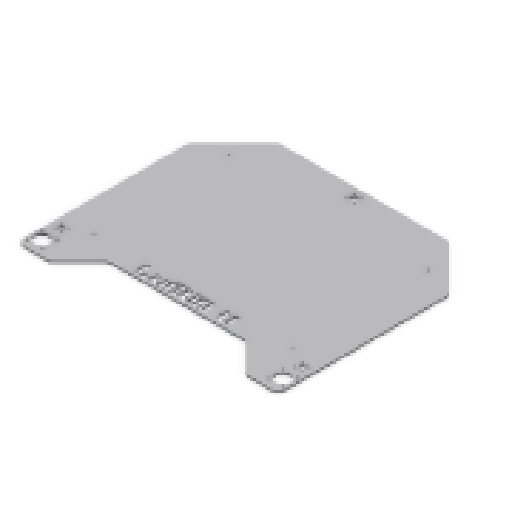
# Autodesk Inventor part: Z Axis Base
Saved by Autodesk Inventor 2023.2 (Build 272271000, 271)
## iProperties
Created: 2023-02-02
Part Number: Z Axis Base
Material: Aluminum 6061
Document SubType Name: Modeling
Designer: remop
Density: 2.7 g/cm^3
Appearance: Aluminum - Dark
Author: remop
Autodesk Inventor part; units mm, degrees
ref_plane "YZ Plane" through (0, 0, 0) normal (1, 0, 0) x (0, 1, 0)
ref_plane "XZ Plane" through (0, 0, 0) normal (0, 1, 0) x (-1, 0, 0)
ref_plane "XY Plane" through (0, 0, 0) normal (0, 0, 1) x (1, 0, 0)
sketch "Sketch1" plane through (0, 0, 0) normal (0, 1, 0) x (-1, 0, 0)
  circle A0 centre (158.2314, 130.3812) radius 11.25 projected
  circle A1 centre (158.2314, 160.3812) radius 6 projected
  circle A2 centre (-213.7686, 130.3812) radius 11.25 projected
  circle A3 centre (-213.7686, 160.3812) radius 6 projected
  circle A4 centre (-27.7686, -135.6188) radius 11 projected
  circle A5 centre (125.7314, 112.8812) radius 1.75
  circle A6 centre (125.7314, -96.1188) radius 1.75
  circle A7 centre (-181.2686, -96.1188) radius 1.75
  circle A8 centre (-181.2686, 112.8812) radius 1.75
  line L0 (222.2314, 188.3812) -> (-277.7686, 188.3812) projected
  line L1 (222.2314, -171.6188) -> (-277.7686, -171.6188) projected
  line L2 (174.2314, 183.3812) -> (124.2314, 183.3812)
  line L3 (124.2314, 183.3812) -> (78.7314, 137.8812)
  line L4 (78.7314, 137.8812) -> (-134.2686, 137.8812)
  line L5 (-134.2686, 137.8812) -> (-179.7686, 183.3812)
  line L6 (-179.7686, 183.3812) -> (-229.7686, 183.3812)
  line L7 (-229.7686, 183.3812) -> (-229.7686, -151.6188)
  line L8 (-229.7686, -151.6188) -> (174.2314, -151.6188)
  line L9 (174.2314, -151.6188) -> (174.2314, 183.3812)
  line L10 (222.2314, -171.6188) -> (222.2314, 188.3812) projected
  line L11 (-277.7686, 188.3812) -> (-277.7686, -171.6188) projected
  circle A9 centre (-213.7686, 160.3812) radius 11.5
  circle A10 centre (-225.2686, 171.8812) radius 2.1
  circle A11 centre (-202.2686, 171.8812) radius 2.1
  circle A12 centre (-202.2686, 148.8812) radius 2.1
  circle A13 centre (-225.2686, 148.8812) radius 2.1
  circle A14 centre (158.2314, 160.3812) radius 11.5
  circle A15 centre (146.7314, 171.8812) radius 2.1
  circle A16 centre (169.7314, 171.8812) radius 2.1
  circle A17 centre (169.7314, 148.8812) radius 2.1
  circle A18 centre (146.7314, 148.8812) radius 2.1
  circle A19 centre (-213.7686, 130.3812) radius 4.5
  circle A20 centre (-219.2686, 124.8812) radius 1.6
  circle A21 centre (-219.2686, 135.8812) radius 1.6
  circle A22 centre (-208.2686, 135.8812) radius 1.6
  circle A23 centre (-208.2686, 124.8812) radius 1.6
  circle A24 centre (158.2314, 130.3812) radius 4.5
  circle A25 centre (152.7314, 135.8812) radius 1.6
  circle A26 centre (163.7314, 135.8812) radius 1.6
  circle A27 centre (163.7314, 124.8812) radius 1.6
  circle A28 centre (152.7314, 124.8812) radius 1.6
  circle A29 centre (-27.7686, -135.6188) radius 4.5
  circle A30 centre (-33.2686, -130.1188) radius 1.6
  circle A31 centre (-22.2686, -130.1188) radius 1.6
  circle A32 centre (-22.2686, -141.1188) radius 1.6
  circle A33 centre (-33.2686, -141.1188) radius 1.6
  point P0 (0, 0)
  point P1 (149.2314, 183.3812)
  dimension "d0" = 307
  dimension "d1" = 209
  dimension "d2" = 3.5
  dimension "d3" = 153.5
  dimension "d4" = 360
  dimension "d5" = 75.5
  dimension "d6" = 5
  dimension "d7" = 48
  dimension "d8" = 20
  dimension "d9" = 48
  dimension "d10" = 5
  dimension "d12" = 45
  dimension "d13" = 50
  dimension "d14" = 45
  dimension "d15" = 25
  dimension "d18" = 23
  dimension "d19" = 11.5
  dimension "d20" = 11.5
  dimension "d21" = 11.5
  dimension "d22" = 11.5
  dimension "d23" = 4.2
  dimension "d24" = 11.5
  dimension "d25" = 11.5
  dimension "d26" = 11.5
  dimension "d27" = 11.5
  dimension "d28" = 9
  dimension "d29" = 5.5
  dimension "d30" = 5.5
  dimension "d31" = 5.5
  dimension "d32" = 5.5
  dimension "d33" = 3.2
  dimension "d35" = 5.5
  dimension "d36" = 5.5
  dimension "d37" = 5.5
  dimension "d39" = 5.5
  dimension "d40" = 5.5
  dimension "d41" = 5.5
  dimension "d42" = 5.5
  dimension "d43" = 5.5
  constraints: 29 centre point, 24 equal radius, 16 end point, 12 horizontal alignment, 12 vertical alignment, 5 coincident, 3 parallel, 1 collinear, 1 horizontal, 1 midpoint, 1 perpendicular
  measures "d0" distance of A8.centre A5.centre
  measures "d1" distance of A6.centre A5.centre
  measures "d2" diameter of A5
  measures "d3" horizontal distance of A6.centre A4.centre
  measures "d4" distance between parallel lines of L1 L0
  measures "d5" distance from line of L1 A7.centre
  measures "d6" distance between parallel lines of L0 L6
  measures "d7" distance between parallel lines of L11 L7
  measures "d8" distance between parallel lines of L1 L8
  measures "d9" distance between parallel lines of L10 L9
  measures "d10" distance from line of L0 point (149.231, 183.381)
  measures "d12" angle of L2 L3
  measures "d13" distance of L2.start L2.end
  measures "d14" angle of L6 L5
  measures "d15" distance from line of A5.centre L4
  measures "d18" diameter of A9
  measures "d19" horizontal distance of A3.centre A10.centre
  measures "d20" horizontal distance of A3.centre A11.centre
  measures "d21" horizontal distance of A10.centre A9.centre
  measures "d22" horizontal distance of A13.centre A3.centre
  measures "d23" diameter of A13
  measures "d24" horizontal distance of A15.centre A1.centre
  measures "d25" horizontal distance of A18.centre A1.centre
  measures "d26" horizontal distance of A1.centre A18.centre
  measures "d27" horizontal distance of A17.centre A14.centre
  measures "d28" diameter of A19
  measures "d29" horizontal distance of A21.centre A2.centre
  measures "d30" horizontal distance of A19.centre A21.centre
  measures "d31" horizontal distance of A22.centre A2.centre
  measures "d32" horizontal distance of A20.centre A2.centre
  measures "d33" diameter of A20
  measures "d35" horizontal distance of A25.centre A0.centre
  measures "d36" horizontal distance of A25.centre A0.centre
  measures "d37" horizontal distance of A0.centre A26.centre
  measures "d39" horizontal distance of A0.centre A28.centre
  measures "d40" horizontal distance of A31.centre A29.centre
  measures "d41" horizontal distance of A30.centre A4.centre
  measures "d42" horizontal distance of A31.centre A29.centre
  measures "d43" horizontal distance of A32.centre A29.centre
extrude "Extrusion1" add sketch "Sketch1" along normal blind 3 contours A0 | A2 | A4 | L9 L8 L7 L6 L5 L4 L3 L2
sketch "Sketch2" plane through (0, 3, 0) normal (0, 1, 0) x (1, 0, 0)
  line L0 (-124.2314, -183.3812) -> (-78.7314, -137.8812) projected
  line L1 (-78.7314, -137.8812) -> (134.2686, -137.8812) projected
  line L2 (134.2686, -137.8812) -> (179.7686, -183.3812) projected
  line L3 (179.7686, -183.3812) -> (229.7686, -183.3812) projected
  line L4 (229.7686, -183.3812) -> (229.7686, 151.6188) projected
  line L5 (229.7686, 151.6188) -> (-174.2314, 151.6188) projected
  line L6 (-174.2314, 151.6188) -> (-174.2314, -183.3812) projected
  line L7 (-174.2314, -183.3812) -> (-124.2314, -183.3812) projected
  circle A0 centre (-158.2314, -130.3812) radius 4.5 projected
  circle A1 centre (-152.7314, -135.8812) radius 1.6 projected
  circle A2 centre (-163.7314, -135.8812) radius 1.6 projected
  circle A3 centre (-163.7314, -124.8812) radius 1.6 projected
  circle A4 centre (-152.7314, -124.8812) radius 1.6 projected
  circle A5 centre (213.7686, -130.3812) radius 4.5 projected
  circle A6 centre (219.2686, -124.8812) radius 1.6 projected
  circle A7 centre (219.2686, -135.8812) radius 1.6 projected
  circle A8 centre (208.2686, -135.8812) radius 1.6 projected
  circle A9 centre (208.2686, -124.8812) radius 1.6 projected
  circle A10 centre (27.7686, 135.6188) radius 4.5 projected
  circle A11 centre (33.2686, 130.1188) radius 1.6 projected
  circle A12 centre (22.2686, 130.1188) radius 1.6 projected
  circle A13 centre (22.2686, 141.1188) radius 1.6 projected
  circle A14 centre (33.2686, 141.1188) radius 1.6 projected
  circle A15 centre (-125.7314, -112.8812) radius 1.75 projected
  circle A16 centre (-125.7314, 96.1188) radius 1.75 projected
  circle A17 centre (181.2686, 96.1188) radius 1.75 projected
  circle A18 centre (181.2686, -112.8812) radius 1.75 projected
  circle A19 centre (-146.7314, -148.8812) radius 2.1 projected
  circle A20 centre (-169.7314, -148.8812) radius 2.1 projected
  circle A21 centre (-169.7314, -171.8812) radius 2.1 projected
  circle A22 centre (-146.7314, -171.8812) radius 2.1 projected
  circle A23 centre (-158.2314, -160.3812) radius 11.5 projected
  circle A24 centre (225.2686, -148.8812) radius 2.1 projected
  circle A25 centre (202.2686, -148.8812) radius 2.1 projected
  circle A26 centre (202.2686, -171.8812) radius 2.1 projected
  circle A27 centre (225.2686, -171.8812) radius 2.1 projected
  circle A28 centre (213.7686, -160.3812) radius 11.5 projected
  line L8 (-71.2064, -116.1262) -> (126.7436, -116.1262) construction
  line L9 (126.7436, -116.1262) -> (126.7436, -129.6362) construction
  line L10 (126.7436, -129.6362) -> (-71.2064, -129.6362) construction
  line L11 (-71.2064, -129.6362) -> (-71.2064, -116.1262) construction
  line L12 (-41.9641, -132.872) -> (-44.5632, -130.2729)
  line L13 (-44.5632, -130.2729) -> (-44.5632, -112.872)
  line L14 (-44.5632, -112.872) -> (-37.5955, -112.872)
  line L15 (-37.5955, -112.872) -> (-37.5955, -132.872)
  line L16 (-37.5955, -132.872) -> (-41.9641, -132.872)
  line L17 (-36.7844, -132.872) -> (-36.7844, -126.9549)
  line L18 (-36.7844, -126.9549) -> (-23.66, -126.9549)
  line L19 (-23.66, -126.9549) -> (-23.66, -132.872)
  line L20 (-23.66, -132.872) -> (-36.7844, -132.872)
  line L21 (-9.3743, -132.8536) -> (-19.3282, -132.8536)
  line L22 (-19.3282, -132.8536) -> (-22.554, -129.6277)
  line L23 (-22.554, -129.6277) -> (-22.554, -118.4388)
  line L24 (-22.554, -118.4388) -> (-15.4941, -118.4388)
  line L25 (-15.4941, -118.4388) -> (-15.4941, -126.9365)
  line L26 (-15.4941, -126.9365) -> (-9.3743, -126.9365)
  line L27 (-9.3743, -126.9365) -> (-9.3743, -132.8536)
  line L28 (-1.5402, -132.8536) -> (-8.6001, -132.8536)
  line L29 (-8.6001, -132.8536) -> (-8.6001, -118.4388)
  line L30 (-8.6001, -118.4388) -> (-1.5402, -118.4388)
  line L31 (-1.5402, -118.4388) -> (-1.5402, -132.8536)
  line L32 (6.5889, -132.872) -> (2.1649, -132.872)
  line L33 (2.1649, -132.872) -> (-0.4342, -130.2729)
  line L34 (-0.4342, -130.2729) -> (-0.4342, -115.4711)
  line L35 (-0.4342, -115.4711) -> (2.1649, -112.872)
  line L36 (2.1649, -112.872) -> (6.5889, -112.872)
  line L37 (6.5889, -112.872) -> (6.5889, -132.872)
  line L38 (20.5797, -119.0471) -> (7.3999, -119.0471)
  line L39 (7.3999, -119.0471) -> (7.3999, -112.872)
  line L40 (7.3999, -112.872) -> (20.5797, -112.872)
  line L41 (20.5797, -112.872) -> (20.5797, -119.0471)
  line L42 (20.5797, -132.872) -> (7.3999, -132.872)
  line L43 (7.3999, -132.872) -> (7.3999, -126.9549)
  line L44 (7.3999, -126.9549) -> (20.5797, -126.9549)
  line L45 (20.5797, -126.9549) -> (20.5797, -132.872)
  line L46 (20.5797, -124.7061) -> (7.3999, -124.7061)
  line L47 (7.3999, -124.7061) -> (7.3999, -119.8582)
  line L48 (7.3999, -119.8582) -> (20.5797, -119.8582)
  line L49 (20.5797, -119.8582) -> (20.5797, -124.7061)
  line L50 (34.8654, -132.8904) -> (28.3216, -132.8904)
  line L51 (28.3216, -132.8904) -> (21.6856, -126.2545)
  line L52 (21.6856, -126.2545) -> (21.6856, -112.872)
  line L53 (21.6856, -112.872) -> (28.7455, -112.872)
  line L54 (28.7455, -112.872) -> (28.7455, -126.5678)
  line L55 (28.7455, -126.5678) -> (34.8654, -126.5678)
  line L56 (34.8654, -126.5678) -> (34.8654, -132.8904)
  line L57 (35.6396, -132.872) -> (35.6396, -112.872)
  line L58 (35.6396, -112.872) -> (42.5889, -112.872)
  line L59 (42.5889, -112.872) -> (42.5889, -126.2176)
  line L60 (42.5889, -126.2176) -> (35.6396, -132.872)
  line L61 (50.7548, -132.872) -> (46.2939, -132.872)
  line L62 (46.2939, -132.872) -> (43.6949, -130.2729)
  line L63 (43.6949, -130.2729) -> (43.6949, -115.4711)
  line L64 (43.6949, -115.4711) -> (46.3124, -112.872)
  line L65 (46.3124, -112.872) -> (56.8746, -112.872)
  line L66 (56.8746, -112.872) -> (56.8746, -119.0471)
  line L67 (56.8746, -119.0471) -> (50.7548, -119.0471)
  line L68 (50.7548, -119.0471) -> (50.7548, -132.872)
  line L69 (64.7087, -130.2545) -> (62.0912, -132.872)
  line L70 (62.0912, -132.872) -> (51.4921, -132.872)
  line L71 (51.4921, -132.872) -> (51.4921, -126.9549)
  line L72 (51.4921, -126.9549) -> (57.6488, -126.9549)
  line L73 (57.6488, -126.9549) -> (57.6488, -112.872)
  line L74 (57.6488, -112.872) -> (62.0912, -112.872)
  line L75 (62.0912, -112.872) -> (64.7087, -115.4895)
  line L76 (64.7087, -115.4895) -> (64.7087, -130.2545)
  line L77 (92.9299, -132.8904) -> (86.3861, -132.8904)
  line L78 (86.3861, -132.8904) -> (79.7502, -126.2545)
  line L79 (79.7502, -126.2545) -> (79.7502, -112.872)
  line L80 (79.7502, -112.872) -> (86.8101, -112.872)
  line L81 (86.8101, -112.872) -> (86.8101, -126.5678)
  line L82 (86.8101, -126.5678) -> (92.9299, -126.5678)
  line L83 (92.9299, -126.5678) -> (92.9299, -132.8904)
  line L84 (93.7041, -132.872) -> (93.7041, -112.872)
  line L85 (93.7041, -112.872) -> (100.6534, -112.872)
  line L86 (100.6534, -112.872) -> (100.6534, -126.2176)
  line L87 (100.6534, -126.2176) -> (93.7041, -132.872)
  point P0 (0, 0)
  point P1 (27.7686, -116.1262)
  point P2 (-71.2064, -122.8812)
  dimension "d44" = 15
  constraints: 2 midpoint, 1 vertical alignment, 2 other
  measures "d44" distance from line of L1 point (-71.206, -122.881)
extrude "Extrusion2" cut sketch "Sketch2" against normal through all contours L12 L13 L14 L15 L16 | L17 L18 L19 L20 | L21 L22 L23 L24 L25 L26 L27 | L28 L29 L30 L31 | L32 L33 L34 L35 L36 L37 | L38 L39 L40 L41 | L42 L43 L44 L45 | L46 L47 L48 L49 | L50 L51 L52 L53 L54 L55 L56 | L57 L58 L59 L60 | L61 L62 L63 L64 L65 L66 L67 L68 | L69 L70 L71 L72 L73 L74 L75 L76 | L77 L78 L79 L80 L81 L82 L83 | L84 L85 L86 L87
sketch "Sketch3" plane through (0, 3, 0) normal (0, 1, 0) x (1, 0, 0)
  line L0 (134.2686, -137.8812) -> (179.7686, -183.3812) projected
  line L1 (229.7686, -183.3812) -> (229.7686, 151.6188) projected
  line L2 (229.7686, 151.6188) -> (-174.2314, 151.6188) projected
  line L3 (-174.2314, 151.6188) -> (-174.2314, -183.3812) projected
  line L4 (-124.2314, -183.3812) -> (-78.7314, -137.8812) projected
  line L5 (-103.5207, 151.6188) -> (-174.2314, 80.9081)
  line L6 (-174.2314, 151.6188) -> (-174.2314, -183.3812) projected
  line L7 (229.7686, 80.9081) -> (159.0579, 151.6188)
  point P0 (0, 0)
  point P1 (-174.2314, 80.9081)
  dimension "d47" = 100
  constraints: 4 end point, 4 point on line, 2 parallel, 1 perpendicular
  measures "d47" distance of L7.start L7.end
extrude "Extrusion3" cut sketch "Sketch3" against normal through all
fillet "Fillet1" radius 10 10 edges at (-174.2314, 1.5, 183.3812) (-124.2314, 1.5, 183.3812) (229.7686, 1.5, 183.3812) (179.7686, 1.5, 183.3812) (134.2686, 1.5, 137.8812) (229.7686, 1.5, -80.9081) (159.0579, 1.5, -151.6188) (-103.5207, 1.5, -151.6188) (-174.2314, 1.5, -80.9081) (-78.7314, 1.5, 137.8812)
equation "\"d3\" = 0.5 * d0"
equation "\"d5\" = 0.5 * d4 - 0.5 * d1"
equation "\"d9\" = d7"
equation "\"d10\" = d6"
equation "\"d14\" = d12"
equation "\"d20\" = d19"
equation "\"d21\" = d19"
equation "\"d22\" = d19"
equation "\"d24\" = d19"
equation "\"d25\" = d24"
equation "\"d26\" = d24"
equation "\"d27\" = d26"
equation "\"d30\" = d29"
equation "\"d31\" = d30"
equation "\"d32\" = d29"
equation "\"d35\" = d29"
equation "\"d36\" = d35"
equation "\"d37\" = d36"
equation "\"d39\" = d35"
equation "\"d40\" = d35"
equation "\"d41\" = d40"
equation "\"d42\" = d40"
equation "\"d43\" = d42"
body "Solid1"
